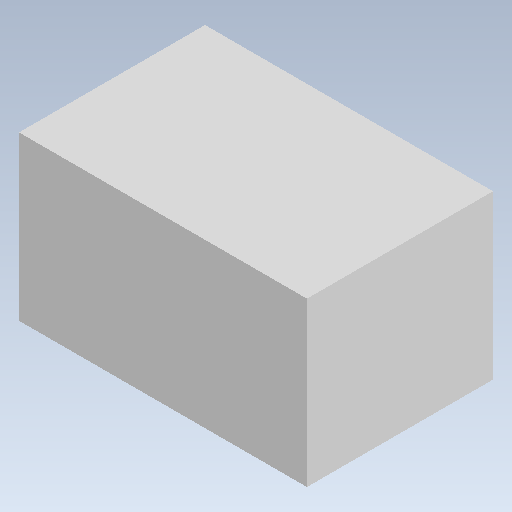
# Autodesk Inventor part: Button_base
Saved by Autodesk Inventor 2020 (Build 240168000, 168)
## iProperties
Created: 2020-08-08
Part Number: Button_base
Material: Generic
Document SubType Name: Modeling
Designer: reide
Density: 1 g/cm^3
Appearance: Default
Author: reide
Autodesk Inventor part; units mm, degrees
ref_plane "YZ Plane" through (0, 0, 0) normal (1, 0, 0) x (0, 1, 0)
ref_plane "XZ Plane" through (0, 0, 0) normal (0, 1, 0) x (-1, 0, 0)
ref_plane "XY Plane" through (0, 0, 0) normal (0, 0, 1) x (1, 0, 0)
sketch "Sketch1" plane through (0, 0, 0) normal (0, 0, 1) x (1, 0, 0)
  line L0 (0, 0) -> (14.125, 0)
  line L1 (14.125, 0) -> (-14.125, 0)
  line L2 (-14.125, 0) -> (-14.125, -8)
  line L3 (-14.125, -8) -> (-14.125, 8)
  line L4 (-14.125, 8) -> (14.125, 8)
  line L5 (14.125, 8) -> (14.125, -8)
  line L6 (14.125, -8) -> (-14.125, -8)
  line L7 (-14.125, -8) -> (-14.125, 8)
  dimension "d0" = 14.125
  dimension "d1" = 28.25
  dimension "d2" = 8
  dimension "d3" = 16
  constraints: 16 end point, 2 horizontal, 2 parallel, 2 perpendicular, 2 point on line
  measures "d0" distance of L0.start L0.end
  measures "d1" distance of L0.end L1.end
  measures "d2" distance of L1.end L2.end
  measures "d3" distance of L2.end L3.end
extrude "Extrusion1" add sketch "Sketch1" along normal blind 18.25
body "Solid1"
